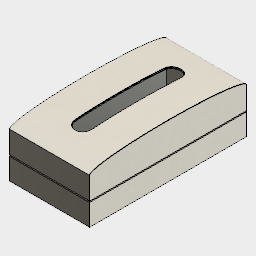
boite a mouchoir (Autodesk Fusion 360 design; units mm, degrees)
Autodesk Fusion 360 part; units mm, degrees
note: some values were not read from the file. Set by a fixed rule: which sketch regions a step uses; which face or edge a step refers to.
sketch "Sketch1" plane through (0, 0, 0) normal (0, 1, 0) x (1, 0, 0)
  line L0 (0, 0) -> (133, 0)
  line L1 (133, 0) -> (133, -260)
  line L2 (133, -260) -> (0, -260)
  line L3 (0, -260) -> (0, 0)
  dimension "d1" = 133
  dimension "d2" = 260
  measures "d1" distance of L0.start L0.end
  measures "d2" distance of L0.start L2.end
extrude "Extrude1" add sketch "Sketch1" along normal blind 47 makes body 1
ref_plane "WorkPlane1" through (66.5, 47, 130) normal (0, 1, 0) x (0, 0, 1)
sketch "Sketch2" plane through (66.5, 47, 130) normal (0, 1, 0) x (1, 0, 0)
  line L0 (-66.5, 130) -> (-66.5, -130)
  line L1 (-66.5, -130) -> (-66.5, 130)
  line L2 (-66.5, 116.0941) -> (-61.5, 116.0941) construction
  line L3 (-66.5, 105.206) -> (-61.5, 105.206) construction
  line L4 (-61.5, 105.206) -> (-61.5, 130)
  line L5 (66.5, 130) -> (-66.5, 130)
  line L6 (-66.5, 130) -> (66.5, 130)
  line L7 (-50, 130) -> (-50, 125) construction
  line L8 (-50, 125) -> (-61.5, 125)
  line L9 (-66.5, -130) -> (66.5, -130)
  line L10 (45, -130) -> (45, -125) construction
  line L11 (66.5, -130) -> (66.5, 130)
  line L12 (66.5, 130) -> (66.5, -130)
  line L13 (66.5, -115.4312) -> (61.5, -115.4312) construction
  line L14 (61.5, -115.4312) -> (61.5, -130)
  line L15 (45, -125) -> (61.5, -125)
  line L16 (-61.5, 125) -> (61.5, 125)
  line L17 (61.5, 125) -> (61.5, -125)
  line L18 (61.5, -125) -> (-61.5, -125)
  line L19 (-61.5, -125) -> (-61.5, 125)
  line L20 (61.5, -119.9744) -> (63, -119.9744) construction
  line L21 (58.0294, -125) -> (58.0294, -126.5) construction
  line L22 (58.0294, -126.5) -> (66.5, -126.5) construction
  line L23 (63, -119.9744) -> (63, -126.5) construction
  line L24 (-61.5, 122.8746) -> (-63, 122.8746) construction
  line L25 (-58.923, 125) -> (-58.923, 126.5) construction
  line L26 (-58.923, 126.5) -> (-66.5, 126.5) construction
  line L27 (-63, 122.8746) -> (-63, 126.5) construction
  line L28 (63, -126.5) -> (-63, -126.5)
  line L29 (-63, -126.5) -> (-63, 126.5)
  line L30 (-63, 126.5) -> (63, 126.5)
  line L31 (63, 126.5) -> (63, -126.5)
  dimension "d6" = 5
  dimension "d7" = 5
  dimension "d8" = 5
  dimension "d9" = 5
  dimension "d10" = 5
  dimension "d13" = 1.5
  dimension "d14" = 1.5
  dimension "d15" = 1.5
  dimension "d16" = 1.5
  measures "d6" distance of L2.start L2.end
  measures "d7" distance of L3.start L3.end
  measures "d8" distance of L7.start L7.end
  measures "d9" distance of L10.start L10.end
  measures "d10" distance of L13.start L13.end
  measures "d13" distance of L20.start L20.end
  measures "d14" distance of L21.start L21.end
  measures "d15" distance of L24.start L24.end
  measures "d16" distance of L25.start L25.end
extrude "Extrude3" cut sketch "Sketch2" against normal blind 10 contours L0 L1 L4 L5 L6 L9 L14 L28 L29 L30 | L4 L5 L6 L9 L11 L12 L14 L28 L30 L31 bodies 1
extrude "Extrude2" cut sketch "Sketch2" against normal blind 40 contours L4 L8 L14 L15 L16 L17 L18 L19 bodies 1
ref_plane "WorkPlane2" through (66.5, 37, 130) normal (0, 1, 0) x (0, 0, 1)
sketch "Sketch3" plane through (66.5, 37, 130) normal (0, 1, 0) x (1, 0, 0)
  line L0 (66.5, -130) -> (-66.5, -130)
  line L1 (-66.5, -130) -> (-66.5, 130)
  line L2 (-66.5, 130) -> (66.5, 130)
  line L3 (66.5, 130) -> (66.5, -130)
  line L4 (-63, 126.5) -> (63, 126.5)
  line L5 (63, 126.5) -> (63, -126.5)
  line L6 (63, -126.5) -> (-63, -126.5)
  line L7 (-63, -126.5) -> (-63, 126.5)
  point P0 (66.5, -130)
  point P1 (-66.5, 130)
  point P2 (-63, 126.5)
  point P3 (63, -126.5)
extrude "Extrude4" add sketch "Sketch3" along normal blind 52 separate body makes body 2
ref_plane "WorkPlane3" through (0, 63, 130) normal (-1, 0, 0) x (0, 0, 1)
sketch "Sketch4" plane through (0, 63, 130) normal (-1, 0, 0) x (0, 0, -1)
  line L0 (-130, 26) -> (-130, -12)
  line L1 (130, 26) -> (130, -12)
  line L2 (-130, -12) -> (130, -12) construction
  ellipse E0 centre (0, -12) end of major axis (-130, -12) minor radius 14
  line L3 (130, -12) -> (-130, -12)
  line L4 (0, 2) -> (0, -26)
  line L5 (130, -26) -> (-130, -26)
  line L6 (-130, -12) -> (-130, -9)
  line L7 (130, -12) -> (130, -9)
  line L8 (130, -9) -> (-130, -9)
  line L9 (0, -26) -> (0, -23)
  ellipse E1 centre (0, -9) end of major axis (130, -9) minor radius 14
  line L10 (-130, -9) -> (130, -9)
  line L11 (0, -23) -> (0, 5)
  line L12 (130, -26) -> (-130, -26)
  line L13 (-130, -26) -> (-130, 26)
  line L14 (-130, 26) -> (130, 26)
  line L15 (130, 26) -> (130, -26)
  point P0 (-130, 26)
  point P1 (130, 26)
  dimension "d23" = 38
  dimension "d24" = 38
  dimension "d25" = 3
  dimension "d26" = 3
  dimension "d27" = 3
  measures "d23" distance of P0 L0.end
  measures "d24" distance of P1 L1.end
  measures "d25" distance of L0.end L6.end
  measures "d26" distance of L1.end L7.end
  measures "d27" distance of L4.end L9.end
extrude "Extrude6" add sketch "Sketch4" against normal up to surface (133 mm away) contours L0 E0 L6 E1 L13 | E0 L3 L4 L9 E1 | E0 L3 E1 | L1 E0 L7 E1 L15 | E0 L3 L4 L9 E1 | E0 L3 E1 bodies 2
extrude "Extrude5" cut sketch "Sketch4" against normal up to surface (133 mm away) contours E0 L5 L12 L13 | E0 L5 L12 L15 bodies 2
ref_plane "WorkPlane4" through (66.5, 97, 130) normal (0, 1, 0) x (0, 0, 1)
sketch "Sketch5" plane through (66.5, 97, 130) normal (0, 1, 0) x (1, 0, 0)
  line L0 (-66.5, 130) -> (66.5, 130)
  line L1 (66.5, 130) -> (66.5, -130)
  line L2 (66.5, -130) -> (-66.5, -130)
  line L3 (-66.5, -130) -> (-66.5, 130)
  line L4 (0, -130) -> (0, -87)
  line L5 (0, 130) -> (0, 87)
  circle A0 centre (0, 73.5) radius 13.5
  circle A1 centre (0, -73.5) radius 13.5
  line L6 (0, 73.5) -> (-66.5, 73.5) construction
  line L7 (0, -73.5) -> (66.5, -73.5) construction
  line L8 (-13.5, 73.5) -> (13.5, 73.5)
  line L9 (13.5, 73.5) -> (13.5, -73.5)
  line L10 (13.5, -73.5) -> (-13.5, -73.5)
  line L11 (-13.5, -73.5) -> (-13.5, 73.5)
  point P0 (-66.5, 130)
  point P1 (66.5, -130)
  dimension "d33" = 43
  dimension "d34" = 43
  dimension "d35" = 27
  dimension "d36" = 27
  measures "d33" distance of L4.start L4.end
  measures "d34" distance of L5.start L5.end
  measures "d35" diameter of A0
  measures "d36" diameter of A1
extrude "Extrude7" cut sketch "Sketch5" along normal up to surface contours A0 L8 | A0 A1 L9 L11 | A0 L8 | A1 L10 | A1 L10 end surface at (87.5, 85.1475, 174.6703) on bodies 2 bodies 2
fillet "Fillet1" radius 1 4 edges at (66.5, 37, 0) (133, 37, 130) (0, 37, 130) (66.5, 37, 260) on bodies 1
fillet "Fillet2" radius 1 4 edges at (0, 37, 130) (66.5, 37, 260) (133, 37, 130) (66.5, 37, 0) on bodies 2
fillet "Fillet3" radius 0.5 7 edges at (133, 18, 0) (132.7071, 36.7071, 0.2929) (132.7071, 37.2929, 0.2929) (133, 56.5, 0) (133, 89, 130) (133, 56.5, 260) (132.7071, 37.2929, 259.7071) on bodies 1 2
fillet "Fillet4" radius 0.5 2 edges at (133, 18, 260) (132.7071, 36.7071, 259.7071) on bodies 1
fillet "Fillet5" radius 0.5 9 edges at (0, 18, 0) (0.2929, 36.7071, 0.2929) (0, 18, 260) (0.2929, 36.7071, 259.7071) (0.2929, 37.2929, 259.7071) (0, 56.5, 260) (0, 89, 130) (0, 56.5, 0) (0.2929, 37.2929, 0.2929) on bodies 1 2
fillet "Fillet6" radius 0.7 8 edges at (53, 89, 130) (66.5, 85.4028, 43) (80, 89, 130) (66.5, 85.4028, 217) (53, 86, 130) (66.5, 82.4028, 217) (80, 86, 130) (66.5, 82.4028, 43) on bodies 2
fillet "Fillet7" radius 0.5 8 edges at (132.8536, 0, 259.8536) (66.5, 0, 260) (0.1464, 0, 259.8536) (0, 0, 130) (0.1464, 0, 0.1464) (66.5, 0, 0) (132.8536, 0, 0.1464) (133, 0, 130) on bodies 1
named bodies: "botom", "cover"
